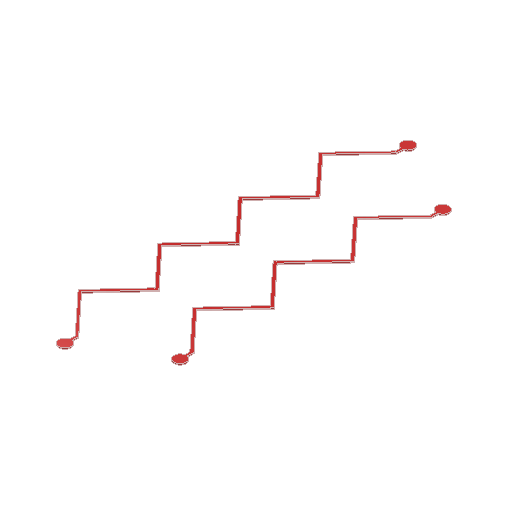
# Autodesk Inventor part: Serpentine
Saved by Autodesk Inventor 2025.4 (Build 294407000, 407)
## iProperties
Created: 2026-04-28
Part Number: Serpentine
Material: Generic
Document SubType Name: Modeling
Designer: gdira
Density: 1 g/cm^3
Appearance: Default
Author: gdira
Autodesk Inventor part; units mm, degrees
ref_plane "YZ Plane" through (0, 0, 0) normal (1, 0, 0) x (0, 1, 0)
ref_plane "XZ Plane" through (0, 0, 0) normal (0, 1, 0) x (-1, 0, 0)
ref_plane "XY Plane" through (0, 0, 0) normal (0, 0, 1) x (1, 0, 0)
sketch "Sketch1" plane through (0, 0, 0) normal (0, 1, 0) x (-1, 0, 0)
  line L0 (-4.3027, -54.4168) -> (-19.3027, -54.4168)
  line L1 (-18.0377, 10.5832) -> (-4.3027, 10.5832)
  line L2 (-18.0418, -21.9168) -> (-4.3027, -21.9168)
  line L3 (-5.8006, -38.3056) -> (-19.5609, -39.5644)
  line L4 (-4.3027, 10.5832) -> (-18.0377, 10.5832)
  line L5 (-5.8333, -5.6668) -> (-19.5609, -4.2692)
  line L6 (-4.4358, 75.5832) -> (-19.3005, 75.5832)
  line L7 (-18.0377, 43.0832) -> (-4.3027, 43.0832)
  line L8 (-5.833, 59.3332) -> (-19.5609, 60.7308)
  line L9 (-5.833, 26.8332) -> (-19.5609, 25.4356)
  line L10 (-19.3027, -54.1295) -> (-4.3027, -38.1668)
  line L11 (-4.3027, -38.1668) -> (-5.0315, -37.482)
  line L12 (-5.8006, -38.3056) -> (-20.3027, -53.7385)
  line L13 (-20.3027, -53.7385) -> (-20.3005, -53.7406)
  line L14 (-4.3027, -38.1668) -> (-18.6745, -22.5975)
  line L15 (-19.568, -21.9168) -> (-20.3028, -22.5951)
  line L16 (-20.3028, -22.5951) -> (-5.8006, -38.3056)
  line L17 (-5.0376, -38.8451) -> (-4.3027, -38.1668)
  line L18 (-20.3028, -22.5951) -> (-5.2007, -6.3475)
  line L19 (-4.3027, -5.6668) -> (-3.5703, -6.3476)
  line L20 (-19.5632, -23.2824) -> (-20.3028, -22.5951)
  line L21 (-3.5703, -6.3476) -> (-18.6702, 9.9025)
  line L22 (-19.568, 10.5832) -> (-20.3005, 9.9025)
  line L23 (-20.3005, 9.9025) -> (-5.2007, -6.3475)
  line L24 (-4.3029, -7.0283) -> (-3.5703, -6.3476)
  line L25 (-20.3005, 9.9025) -> (-5.2005, 26.1525)
  line L26 (-4.3027, 26.8332) -> (-3.5702, 26.1525)
  line L27 (-3.5702, 26.1525) -> (-18.6702, 9.9025)
  line L28 (-19.568, 9.2218) -> (-20.3005, 9.9025)
  line L29 (-3.5702, 26.1525) -> (-18.6702, 42.4025)
  line L30 (-19.568, 43.0832) -> (-20.3005, 42.4025)
  line L31 (-20.3005, 42.4025) -> (-5.2005, 26.1525)
  line L32 (-4.3027, 25.4718) -> (-3.5702, 26.1525)
  line L33 (-20.3005, 42.4025) -> (-5.2009, 58.653)
  line L34 (-4.4358, 59.1909) -> (-3.7033, 58.5103)
  line L35 (-3.7033, 58.5103) -> (-18.6702, 42.4025)
  line L36 (-19.568, 41.7218) -> (-20.3005, 42.4025)
  line L37 (-3.7033, 58.5103) -> (-19.3005, 75.2954)
  line L38 (-20.3005, 74.9025) -> (-5.2009, 58.653)
  line L39 (-4.3027, 57.9718) -> (-3.7033, 58.5103)
  line L40 (-19.5679, -53.7385) -> (-19.3027, -53.7385)
  line L41 (-19.3027, -53.7385) -> (-19.3027, -56.289)
  line L42 (-20.3027, -56.289) -> (-20.3027, -53.7385)
  line L43 (-19.3027, 74.9025) -> (-19.3005, 74.9025)
  line L44 (-19.3005, 75.2954) -> (-19.3005, 77.453)
  line L45 (-20.3005, 77.453) -> (-20.3005, 74.9025)
  arc A0 (-19.3005, 77.453) -> (-20.3005, 77.453) centre (-19.8005, 79.9025) ccw
  arc A1 (-20.3027, -56.289) -> (-19.3027, -56.289) centre (-19.8027, -58.7385) ccw
  line L46 (-19.3027, -58.7385) -> (-19.5679, -58.7385)
  line L47 (-20.3005, -58.7385) -> (-20.3028, -58.7385)
  line L48 (-3.5703, -6.3476) -> (-18.6745, -22.5975)
  line L49 (-19.5609, -23.2799) -> (-19.5632, -23.2824)
  line L50 (-4.3027, -7.0282) -> (-4.3027, -54.4168)
  line L51 (-19.568, -21.9168) -> (-19.568, 9.2218)
  line L52 (-4.3027, 25.4718) -> (-4.3027, -5.6668)
  line L53 (-19.568, 10.5832) -> (-19.568, 41.7218)
  line L54 (-19.568, 43.0832) -> (-19.568, 74.1142)
  line L55 (-4.4358, 75.5832) -> (-4.4358, 59.1909)
  line L56 (-4.3027, 57.9718) -> (-4.3027, 26.8332)
  line L57 (-19.3005, 79.9025) -> (-19.3027, 79.9025)
  line L58 (-19.5609, -52.949) -> (-19.5609, -23.2799)
  line L59 (-33.8119, -38.9953) -> (-48.8119, -38.9953)
  line L60 (-47.5468, 26.0047) -> (-33.8119, 26.0047)
  line L61 (-47.5509, -6.4953) -> (-33.8119, -6.4953)
  line L62 (-35.3097, -22.8842) -> (-49.07, -24.1429)
  line L63 (-33.8119, 26.0047) -> (-47.5468, 26.0047)
  line L64 (-35.3424, 9.7546) -> (-49.07, 11.1522)
  line L65 (-35.3422, 42.2547) -> (-49.07, 40.8571)
  line L66 (-48.8119, -38.708) -> (-33.8119, -22.7453)
  line L67 (-33.8119, -22.7453) -> (-34.5406, -22.0605)
  line L68 (-35.3097, -22.8842) -> (-49.8119, -38.317)
  line L69 (-49.8119, -38.317) -> (-49.8096, -38.3191)
  line L70 (-33.8119, -22.7453) -> (-48.1836, -7.176)
  line L71 (-49.0771, -6.4953) -> (-49.8119, -7.1736)
  line L72 (-49.8119, -7.1736) -> (-35.3097, -22.8842)
  line L73 (-34.5467, -23.4236) -> (-33.8119, -22.7453)
  line L74 (-49.8119, -7.1736) -> (-34.7099, 9.0739)
  line L75 (-33.8119, 9.7547) -> (-33.0794, 9.0739)
  line L76 (-49.0724, -7.861) -> (-49.8119, -7.1736)
  line L77 (-33.0794, 9.0739) -> (-48.1793, 25.324)
  line L78 (-49.0771, 26.0047) -> (-49.8096, 25.324)
  line L79 (-49.8096, 25.324) -> (-34.7099, 9.0739)
  line L80 (-33.812, 8.3932) -> (-33.0794, 9.0739)
  line L81 (-49.8096, 25.324) -> (-34.7096, 41.574)
  line L82 (-33.8119, 42.2547) -> (-33.0793, 41.574)
  line L83 (-33.0793, 41.574) -> (-48.1793, 25.324)
  line L84 (-49.0771, 24.6433) -> (-49.8096, 25.324)
  line L85 (-33.0793, 41.574) -> (-48.1793, 57.824)
  line L86 (-49.8096, 57.8239) -> (-34.7096, 41.574)
  line L87 (-33.8119, 40.8932) -> (-33.0793, 41.574)
  line L88 (-49.0771, -38.317) -> (-48.8119, -38.317)
  line L89 (-48.8119, -38.317) -> (-48.8119, -40.8676)
  line L90 (-49.8119, -40.8676) -> (-49.8119, -38.317)
  arc A2 (-49.8119, -40.8676) -> (-48.8119, -40.8676) centre (-49.3119, -43.317) ccw
  line L91 (-48.8119, -43.317) -> (-49.0771, -43.317)
  line L92 (-49.8096, -43.3171) -> (-49.8119, -43.3171)
  line L93 (-33.0794, 9.0739) -> (-48.1836, -7.176)
  line L94 (-49.07, -7.8585) -> (-49.0724, -7.861)
  line L95 (-33.8119, 8.3932) -> (-33.8119, -38.9953)
  line L96 (-49.0771, -6.4953) -> (-49.0771, 24.6433)
  line L97 (-33.8119, 40.8932) -> (-33.8119, 9.7547)
  line L98 (-49.0771, 26.0047) -> (-49.0771, 57.1433)
  line L99 (-33.8119, 73.3932) -> (-33.8119, 42.2547)
  line L100 (-49.07, -37.5276) -> (-49.07, -7.8585)
  line L101 (-49.0771, 57.1433) -> (-48.8119, 57.1433)
  line L102 (-48.0771, 57.1433) -> (-48.0771, 62.1433)
  line L103 (-48.0771, 62.1433) -> (-49.0771, 62.1433)
  line L104 (-49.0771, 62.1433) -> (-49.0771, 57.1433)
  circle A3 centre (-48.5771, 62.1433) radius 2.5
  point P0 (0, 0)
  point P1 (-4.3027, 59.3332)
  point P2 (-4.3027, -7.1356)
  point P3 (-4.3027, -5.5594)
  point P4 (-4.3027, 25.3642)
  point P5 (-4.3027, 26.9408)
  point P6 (-4.3027, 57.8651)
  point P7 (-4.4358, 59.2986)
  point P8 (-19.568, 43.1909)
  point P9 (-19.568, 41.6141)
  point P10 (-19.568, 10.6909)
  point P11 (-19.568, 9.1142)
  point P12 (-19.568, -21.8045)
  point P13 (-19.5609, -23.3987)
  point P14 (-33.8119, 8.2858)
  point P15 (-33.8119, 9.8621)
  point P16 (-33.8119, 40.7856)
  point P17 (-33.8119, 42.3623)
  point P18 (-48.0771, 57.7139)
  point P19 (-48.0771, 59.6938)
  point P20 (-49.0771, 59.6938)
  point P21 (-49.0771, 57.0356)
  point P22 (-49.0771, 26.1123)
  point P23 (-49.0771, 24.5356)
  point P24 (-49.0771, -6.3831)
  point P25 (-49.07, -7.9773)
  point P26 (-19.8005, 82.4025)
  point P27 (-19.8027, -61.2385)
  point P28 (-49.3119, -45.817)
  dimension "d0" = 15
  dimension "d2" = 1
  dimension "d3" = 1
  dimension "d4" = 1
  dimension "d5" = 1
  dimension "d6" = 1
  dimension "d7" = 1
  dimension "d8" = 1
  dimension "d10" = 1
  dimension "d11" = 5
  dimension "d12" = 1
  dimension "d13" = 5
  dimension "d14" = 5
  dimension "d15" = 5
  dimension "d18" = 15
  dimension "d19" = 1
  dimension "d20" = 1
  dimension "d21" = 1
  dimension "d22" = 1
  dimension "d23" = 1
  dimension "d26" = 1
  dimension "d27" = 5
  dimension "d31" = 5
  dimension "d32" = 1
  dimension "d33" = 5
  dimension "d34" = 5
  dimension "d35" = 143.641
  dimension "d36" = 107.9603
  constraints: 210 end point, 63 parallel, 34 point on line, 32 perpendicular, 12 symmetric about line, 9 point on circle, 4 centre point, 1 horizontal, 1 midpoint
  measures "d0" distance of L0.start L0.end
  measures "d2" distance of L11.end L10.end
  measures "d3" distance of L15.end L15.start
  measures "d4" distance of L19.start L19.end
  measures "d5" distance of L22.end L22.start
  measures "d6" distance of L26.start L26.end
  measures "d7" distance of L30.end L30.start
  measures "d8" distance of L34.start L34.end
  measures "d10" distance of L12.end L40.end
  measures "d11" distance of L40.end L46.start
  measures "d12" distance of L38.start L43.end
  measures "d13" distance of L57.start L43.end
  measures "d14" diameter of A0
  measures "d15" diameter of A1
  measures "d18" distance of L59.start L59.end
  measures "d19" distance of L67.end L66.end
  measures "d20" distance of L76.end L71.start
  measures "d21" distance of L97.end L75.end
  measures "d22" distance of L78.end L78.start
  measures "d23" distance of L82.start L83.start
  measures "d26" distance of L69.start L88.end
  measures "d27" distance of L88.end L91.start
  measures "d31" diameter of A2
  measures "d32" distance of L98.end L102.start
  measures "d33" distance of L102.end L102.start
  measures "d34" diameter of A3
  measures "d35" distance of point (-19.801, 82.402) point (-19.803, -61.239)
  measures "d36" vertical distance of A3.centre point (-49.312, -45.817)
extrude "Extrusion1" add sketch "Sketch1" along normal blind 0.5 contours L41 A1 L42 L12 L16 L58 L49 L20 L15 L51 L18 L23 L28 L22 L53 L25 L31 L36 L30 L54 L33 L38 L45 A0 L44 L37 L55 L34 L39 L56 L35 L29 L26 L32 L52 L27 L21 L19 L24 L50 L48 L14 L10 | L89 A2 L90 L68 L72 L100 L94 L76 L71 L96 L74 L79 L84 L78 L98 L81 L86 L104 A3 L102 L85 L99 L82 L87 L97 L83 L77 L75 L80 L95 L93 L70 L66 | A3 L104 L103 L102 | L102 L103 L104 A3
body "Solid1"
